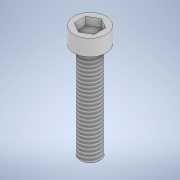
# Autodesk Inventor part: screwM2-5
Saved by Autodesk Inventor 2021 (Build 250183000, 183)
## iProperties
Created: 2021-03-27
Part Number: screwM2-5
Material: Generic
Document SubType Name: Modeling
Designer: lobato
Density: 1 g/cm^3
Appearance: Default
Author: lobato
Autodesk Inventor part; units mm, degrees
ref_plane "YZ Plane" through (0, 0, 0) normal (1, 0, 0) x (0, 1, 0)
ref_plane "XZ Plane" through (0, 0, 0) normal (0, 1, 0) x (-1, 0, 0)
ref_plane "XY Plane" through (0, 0, 0) normal (0, 0, 1) x (1, 0, 0)
sketch "Sketch1" plane through (0, 0, 0) normal (0, 1, 0) x (-1, 0, 0)
  circle A0 centre (0, 0) radius 2
  dimension "d0" = 4
  constraints: 1 centre point, 1 coincident
  measures "d0" diameter of A0
extrude "Extrusion1" add sketch "Sketch1" along normal blind 2
sketch "Sketch2" plane through (0, 0, 0) normal (0, -1, 0) x (1, 0, 0)
  circle A0 centre (0, 0) radius 1.25
  dimension "d3" = 2.5
  constraints: 1 centre point, 1 coincident
  measures "d3" diameter of A0
extrude "Extrusion2" add sketch "Sketch2" along normal blind 12
thread "Thread1" size "M2.5x0.45" class "6g" standard "ANSI Metric M Profile" full length
sketch "Sketch3" plane through (0, 2, 0) normal (0, 1, 0) x (1, 0, 0)
  circle A0 centre (0, 0) radius 1.25 projected
  line L0 (0.0005, 1.4434) -> (1.2502, 0.7213)
  line L1 (1.2502, 0.7213) -> (1.2498, -0.7221)
  line L2 (1.2498, -0.7221) -> (-0.0005, -1.4434)
  line L3 (-0.0005, -1.4434) -> (-1.2502, -0.7213)
  line L4 (-1.2502, -0.7213) -> (-1.2498, 0.7221)
  line L5 (-1.2498, 0.7221) -> (0.0005, 1.4434)
  point P0 (-0.6247, 1.0827)
  constraints: 12 end point, 1 coincident, 1 midpoint, 15 other
extrude "Extrusion3" cut sketch "Sketch3" against normal blind 1
body "Solid1"
